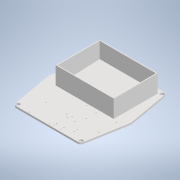
# Autodesk Inventor part: upper base
Saved by Autodesk Inventor 2021 (Build 250183000, 183)
## iProperties
Created: 2021-11-25
Part Number: upper base
Material: Generic
Document SubType Name: Modeling
Designer: techv
Density: 1 g/cm^3
Appearance: Default
Author: techv
Autodesk Inventor part; units mm, degrees
ref_plane "YZ Plane" through (0, 0, 0) normal (1, 0, 0) x (0, 1, 0)
ref_plane "XZ Plane" through (0, 0, 0) normal (0, 1, 0) x (-1, 0, 0)
ref_plane "XY Plane" through (0, 0, 0) normal (0, 0, 1) x (1, 0, 0)
sketch "Sketch1" plane through (0, 0, 0) normal (0, 1, 0) x (-1, 0, 0)
  arc A0 (-85.6318, 54.0093) -> (-85.4518, 52.6798) centre (-90.4518, 52.6798) ccw projected
  line L0 (-85.6318, 54.0093) -> (-85.6318, 82.6798) projected
  line L1 (-85.6318, 82.6798) -> (-75.8236, 82.6798) projected
  line L2 (-75.8236, 82.6798) -> (-75.8236, 52.6798) projected
  line L3 (-75.8236, 52.6798) -> (-85.4518, 52.6798) projected
  circle A1 centre (89.5482, 282.6798) radius 5 projected
  circle A2 centre (-90.4518, 282.6798) radius 5 projected
  circle A3 centre (89.5482, 52.6798) radius 5 projected
  circle A4 centre (-15.4518, 247.6798) radius 5 projected
  circle A5 centre (94.5482, 87.6798) radius 5 projected
  circle A6 centre (-15.4518, 87.6798) radius 5 projected
  circle A7 centre (14.5482, 247.6798) radius 5 projected
  circle A8 centre (-95.4518, 247.6798) radius 5 projected
  circle A9 centre (14.5482, 87.6798) radius 5 projected
  circle A10 centre (-95.4518, 87.6798) radius 5 projected
  circle A11 centre (94.5482, 247.6798) radius 5 projected
  line L4 (-25.6318, 52.6798) -> (-35.3318, 52.6798) projected
  line L5 (-35.3318, 52.6798) -> (-35.3318, 82.6798) projected
  line L6 (-35.3318, 82.6798) -> (-25.6318, 82.6798) projected
  line L7 (-25.6318, 82.6798) -> (-25.6318, 52.6798) projected
  line L8 (24.3682, 82.6798) -> (34.1764, 82.6798) projected
  line L9 (34.1764, 82.6798) -> (34.1764, 52.6798) projected
  line L10 (34.1764, 52.6798) -> (24.3682, 52.6798) projected
  line L11 (24.3682, 52.6798) -> (24.3682, 82.6798) projected
  line L12 (84.3682, 52.6798) -> (74.6682, 52.6798) projected
  line L13 (74.6682, 52.6798) -> (74.6682, 82.6798) projected
  line L14 (74.6682, 82.6798) -> (84.3682, 82.6798) projected
  line L15 (84.3682, 82.6798) -> (84.3682, 52.6798) projected
  arc A12 (86.1572, 45.1798) -> (96.0053, 53.4434) centre (86.1572, 55.1798) ccw projected
  line L16 (96.0053, 53.4434) -> (115.8421, 165.9434) projected
  arc A13 (115.8421, 165.9434) -> (115.8421, 169.4163) centre (105.994, 167.6798) ccw projected
  line L17 (115.8421, 169.4163) -> (96.0053, 281.9163) projected
  arc A14 (96.0053, 281.9163) -> (86.1572, 290.1798) centre (86.1572, 280.1798) ccw projected
  line L18 (86.1572, 290.1798) -> (-87.0608, 290.1798) projected
  arc A15 (-87.0608, 290.1798) -> (-96.9089, 281.9163) centre (-87.0608, 280.1798) ccw projected
  line L19 (-96.9089, 281.9163) -> (-116.7457, 169.4163) projected
  arc A16 (-116.7457, 169.4163) -> (-116.7457, 165.9434) centre (-106.8976, 167.6798) ccw projected
  line L20 (-116.7457, 165.9434) -> (-96.9089, 53.4434) projected
  arc A17 (-96.9089, 53.4434) -> (-87.0608, 45.1798) centre (-87.0608, 55.1798) ccw projected
  line L21 (-87.0608, 45.1798) -> (86.1572, 45.1798) projected
  line L22 (12.0482, 180.1798) -> (12.0482, 155.1798) projected
  line L23 (12.0482, 155.1798) -> (-12.9518, 155.1798) projected
  line L24 (-12.9518, 155.1798) -> (-12.9518, 180.1798) projected
  line L25 (-12.9518, 180.1798) -> (12.0482, 180.1798) projected
  circle A18 centre (25.0482, 100.1798) radius 1.5 projected
  circle A19 centre (25.0482, 230.1798) radius 1.5 projected
  circle A20 centre (-86.9518, 230.1798) radius 1.5 projected
  circle A21 centre (-25.9518, 149.1798) radius 1.5 projected
  circle A22 centre (-25.9518, 100.1798) radius 1.5 projected
  line L26 (-22.4518, 167.6798) -> (-22.4518, 162.6798) projected
  line L27 (-22.4518, 162.6798) -> (-90.4518, 162.6798) projected
  line L28 (-90.4518, 162.6798) -> (-90.4518, 167.6798) projected
  line L29 (-90.4518, 167.6798) -> (-22.4518, 167.6798) projected
  circle A23 centre (-25.9518, 230.1798) radius 1.5 projected
  circle A24 centre (25.0482, 181.1798) radius 1.5 projected
  circle A25 centre (25.0482, 149.1798) radius 1.5 projected
  circle A26 centre (86.0482, 100.1798) radius 1.5 projected
  circle A27 centre (86.0482, 230.1798) radius 1.5 projected
  circle A28 centre (-86.9518, 181.1798) radius 1.5 projected
  circle A29 centre (-86.9518, 149.1798) radius 1.5 projected
  circle A30 centre (-86.9518, 100.1798) radius 1.5 projected
  circle A31 centre (-25.9518, 181.1798) radius 1.5 projected
  line L30 (89.5482, 167.6798) -> (89.5482, 162.6798) projected
  line L31 (89.5482, 162.6798) -> (21.5482, 162.6798) projected
  line L32 (21.5482, 162.6798) -> (21.5482, 167.6798) projected
  line L33 (21.5482, 167.6798) -> (89.5482, 167.6798) projected
  circle A32 centre (86.0482, 181.1798) radius 1.5 projected
  circle A33 centre (86.0482, 149.1798) radius 1.5 projected
  circle A34 centre (-65.4518, 267.6798) radius 4 projected
  circle A35 centre (-65.4518, 67.6798) radius 4 projected
  circle A36 centre (64.5482, 267.6798) radius 4 projected
  circle A37 centre (64.5482, 67.6798) radius 4 projected
  point P0 (0, 0)
extrude "Extrusion1" add sketch "Sketch1" along normal blind 5 contours L0 L1 L2 L3 A0 | A1 | A2 | A3 | A4 | A5 | A6 | A7 | A8 | A9 | A10 | A11 | L4 L5 L6 L7 | L8 L9 L10 L11 | L12 L13 L14 L15 | L21 A17 L20 A16 L19 A15 L18 A14 L17 A13 L16 A12 | L22 L23 L24 L25 | A18 | A19 | A20 | A21 | A22 | L26 L27 L28 L29 | A23 | A24 | A25 | A26 | A27 | A28 | A29 | A30 | A31 | L30 L31 L32 L33 | A32 | A33 | A34 | A35 | A36 | A37
sketch "Sketch2" plane through (0, 5, 0) normal (0, 1, 0) x (1, 0, 0)
  arc A0 (85.6318, -54.0093) -> (85.4518, -52.6798) centre (90.4518, -52.6798) ccw projected
  circle A1 centre (90.4518, -282.6798) radius 5 projected
  circle A2 centre (-89.5482, -52.6798) radius 5 projected
  circle A3 centre (-89.5482, -282.6798) radius 5 projected
  circle A4 centre (90.4518, -52.6798) radius 5
  point P0 (0, 0)
  constraints: 1 centre point, 1 coincident, 1 concentric
extrude "Extrusion2" cut sketch "Sketch2" against normal through all
sketch "Sketch3" plane through (0, 5, 0) normal (0, 1, 0) x (1, 0, 0)
  line L0 (12.9518, -180.1798) -> (12.9518, -155.1798) projected
  line L1 (12.9518, -155.1798) -> (-12.0482, -155.1798) projected
  line L2 (-12.0482, -155.1798) -> (-12.0482, -180.1798) projected
  line L3 (-12.0482, -180.1798) -> (12.9518, -180.1798) projected
  point P0 (0, 0)
extrude "Extrusion3" cut sketch "Sketch3" against normal mid plane 50
sketch "Sketch4" plane through (0, 5, 0) normal (0, 1, 0) x (1, 0, 0)
  line L0 (-12.0482, -155.1798) -> (-12.0482, -180.1798) projected
  line L1 (-12.0482, -180.1798) -> (82.9518, -180.1798)
  line L2 (82.9518, -180.1798) -> (82.9518, -60.1798)
  line L3 (82.9518, -60.1798) -> (-12.0482, -60.1798)
  line L4 (-12.0482, -60.1798) -> (-12.0482, -180.1798)
  line L5 (12.9518, -180.1798) -> (12.9518, -155.1798) projected
  line L6 (12.9518, -180.1798) -> (-82.0482, -180.1798)
  line L7 (-82.0482, -180.1798) -> (-82.0482, -60.1798)
  line L8 (-82.0482, -60.1798) -> (12.9518, -60.1798)
  line L9 (12.9518, -60.1798) -> (12.9518, -180.1798)
  line L10 (82.9518, -60.1798) -> (-82.0482, -60.1798)
  line L11 (-82.0482, -60.1798) -> (-82.0482, -57.6798)
  line L12 (-82.0482, -57.6798) -> (82.9518, -57.6798)
  line L13 (82.9518, -57.6798) -> (82.9518, -60.1798)
  line L14 (-82.0482, -57.6798) -> (-79.5482, -57.6798)
  line L15 (-79.5482, -57.6798) -> (-79.5482, -180.1798)
  line L16 (-79.5482, -180.1798) -> (-82.0482, -180.1798)
  line L17 (-82.0482, -180.1798) -> (-82.0482, -57.6798)
  line L18 (82.9518, -180.1798) -> (80.4518, -180.1798)
  line L19 (80.4518, -180.1798) -> (80.4518, -57.6798)
  line L20 (80.4518, -57.6798) -> (82.9518, -57.6798)
  line L21 (82.9518, -57.6798) -> (82.9518, -180.1798)
  line L22 (82.9518, -180.1798) -> (-82.0482, -180.1798)
  line L23 (-82.0482, -180.1798) -> (-82.0482, -182.6798)
  line L24 (-82.0482, -182.6798) -> (82.9518, -182.6798)
  line L25 (82.9518, -182.6798) -> (82.9518, -180.1798)
  point P0 (0, 0)
  point P1 (-79.5482, -60.1798)
  point P2 (-12.0482, -60.1798)
  point P3 (80.4518, -60.1798)
  dimension "d6" = 95
  dimension "d7" = 120
  dimension "d8" = 95
  dimension "d9" = 120
  dimension "d10" = 2.5
  dimension "d11" = 2.5
  dimension "d12" = 2.5
  dimension "d13" = 2.5
  constraints: 48 end point, 12 parallel, 6 horizontal, 6 perpendicular, 3 point on line
  measures "d6" distance of L3.end L2.end
  measures "d7" distance of L2.end L1.end
  measures "d8" distance of L7.end L8.end
  measures "d9" distance of L6.end L7.end
  measures "d10" distance of L10.end L11.end
  measures "d11" distance of L15.end L16.end
  measures "d12" distance of L19.end L20.end
  measures "d13" distance of L23.end L22.end
extrude "Extrusion4" add sketch "Sketch4" along normal blind 50 contours L1 L25 L24 L23 L6 | L8 L15 L12 L19 L3 | L6 L7 L8 L15 | L8 L11 L12 L15 | L19 L3 L2 L1 | L19 L12 L13 L3
sketch "Sketch6" plane through (80.4518, 5, 60.1798) normal (-1, 0, 0) x (0, 0, 1)
  line L0 (122.5, 0) -> (0, 0) projected
  line L1 (122.5, 0) -> (122.5, 50) projected
  line L2 (0, 50) -> (122.5, 50) projected
  line L3 (0, 0) -> (0, 50) projected
  line L4 (120, 0) -> (120, 50) projected
  line L5 (0, 0) -> (0, 50) projected
  line L6 (0, 0) -> (120, 0)
  line L7 (120, 0) -> (120, 5)
  line L8 (120, 5) -> (0, 5)
  line L9 (0, 5) -> (0, 0)
  line L10 (0, 5) -> (120, 0)
  point P0 (-60.1798, -5)
  dimension "d26" = 5
  constraints: 10 end point, 2 parallel, 1 horizontal, 1 perpendicular, 1 point on line
  measures "d26" distance of L7.end L6.end
extrude "Extrusion6" add sketch "Sketch6" along normal up to surface (160 mm away) contours L0 L3 L10
sketch "Sketch7" plane through (-79.5482, 10, 60.1798) normal (0, 0.9991, 0.0416) x (1, 0, 0)
  line L0 (67.5, -120.1041) -> (67.5, -95.1258) projected
  line L1 (67.5, -95.1258) -> (92.5, -95.1258) projected
  line L2 (92.5, -95.1258) -> (92.5, -120.1041) projected
  line L3 (160, -118.0226) -> (0, -118.0226) projected
  point P0 (79.5482, 59.7114)
  point P1 (67.5, -118.0226)
  point P2 (92.5, -118.0226)
extrude "Extrusion7" cut sketch "Sketch7" against normal blind 10
sketch "Sketch8" plane through (-86.1572, 0, 290.1798) normal (0, 0, 1) x (1, 0, 0)
  line L0 (0, 0) -> (173.218, 0) projected
  line L1 (173.218, 0) -> (173.218, 5) projected
  line L2 (0, 5) -> (173.218, 5) projected
  line L3 (0, 0) -> (0, 5) projected
  line L4 (173.218, 0) -> (173.218, 5) projected
  line L5 (173.218, 0) -> (115.5513, 0)
  line L6 (115.5513, 0) -> (57.8843, 0)
  line L7 (0, 0) -> (173.218, 0) projected
  line L8 (0, 0) -> (-9.8481, 0) projected
  line L9 (0, 0) -> (57.667, 0)
  line L10 (57.667, 0) -> (57.667, 5)
  line L11 (0, 5) -> (173.218, 5) projected
  line L12 (115.5513, 0) -> (115.5513, 5)
  line L13 (99.109, 5) -> (166.609, 5) projected
  line L14 (55.167, 7.5) -> (60.167, 7.5)
  line L15 (60.167, 7.5) -> (60.167, 2.5)
  line L16 (60.167, 2.5) -> (55.167, 2.5)
  line L17 (55.167, 2.5) -> (55.167, 7.5)
  line L18 (55.167, 7.5) -> (60.167, 2.5) construction
  line L19 (60.167, 7.5) -> (55.167, 2.5) construction
  line L20 (113.0513, 7.5) -> (118.0513, 7.5)
  line L21 (118.0513, 7.5) -> (118.0513, 2.5)
  line L22 (118.0513, 2.5) -> (113.0513, 2.5)
  line L23 (113.0513, 2.5) -> (113.0513, 7.5)
  line L24 (113.0513, 7.5) -> (118.0513, 2.5) construction
  line L25 (118.0513, 7.5) -> (113.0513, 2.5) construction
  line L26 (60.167, 2.5) -> (62.667, 2.5)
  line L27 (62.667, 2.5) -> (60.167, 5)
  line L28 (55.167, 2.5) -> (52.667, 2.5)
  line L29 (52.667, 2.5) -> (55.167, 5)
  line L30 (118.0513, 2.5) -> (120.5513, 2.5)
  line L31 (120.5513, 2.5) -> (118.0513, 5)
  line L32 (113.0513, 2.5) -> (110.5513, 2.5)
  line L33 (110.5513, 2.5) -> (113.0513, 5)
  point P0 (86.1572, 0)
  dimension "d31" = 57.6667
  dimension "d33" = 57.667
  dimension "d34" = 5
  dimension "d35" = 5
  dimension "d36" = 5
  dimension "d37" = 5
  dimension "d38" = 2.5
  dimension "d39" = 2.5
  dimension "d40" = 2.5
  dimension "d41" = 2.5
  constraints: 50 end point, 8 midpoint, 6 point on line, 5 horizontal, 4 parallel, 4 perpendicular
  measures "d31" distance of L0.end L5.end
  measures "d33" distance of L0.start L9.end
  measures "d34" distance of L15.end L16.end
  measures "d35" distance of L14.end L15.end
  measures "d36" distance of L21.end L22.end
  measures "d37" distance of L20.end L21.end
  measures "d38" distance of L15.end L26.end
  measures "d39" distance of L16.end L28.end
  measures "d40" distance of L21.end L30.end
  measures "d41" distance of L22.end L32.end
extrude "Extrusion8" cut sketch "Sketch8" against normal up to surface (107.5 mm away) contours L16 L17 L2 L10 | L10 L2 L15 L16 | L17 L28 L29 | L15 L27 L26 | L22 L23 L2 L12 | L12 L2 L21 L22 | L21 L31 L30 | L32 L33 L23
body "Solid1"
